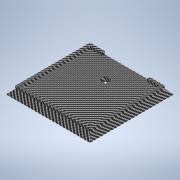
# Autodesk Inventor part: Base Plate
Saved by Autodesk Inventor 2021.1 (Build 251245010, 245A)
## iProperties
Created: 2020-11-23
Part Number: Base Plate
Material: CFRP
Document SubType Name: Modeling
Designer: elizh
Density: 1.43 g/cm^3
Appearance: Carbon Fiber
Author: elizh
Autodesk Inventor part; units mm, degrees
ref_plane "YZ Plane" through (0, 0, 0) normal (1, 0, 0) x (0, 1, 0)
ref_plane "XZ Plane" through (0, 0, 0) normal (0, 1, 0) x (-1, 0, 0)
ref_plane "XY Plane" through (0, 0, 0) normal (0, 0, 1) x (1, 0, 0)
sketch "Sketch1" plane through (0, 0, 0) normal (0, 1, 0) x (-1, 0, 0)
  line L0 (45, 45) -> (-45, 45)
  line L1 (-45, 45) -> (-45, -45)
  line L2 (-45, -45) -> (45, -45)
  line L3 (45, -45) -> (45, 45)
  line L4 (0, 0) -> (55.2623, 0) construction
  line L5 (0, 0) -> (0, -72.148) construction
  dimension "d0" = 90
  constraints: 12 end point, 2 horizontal, 2 parallel, 2 perpendicular, 1 vertical, 2 other
  measures "d0" distance of L2.end L0.start
extrude "Extrusion1" add sketch "Sketch1" along normal blind 5
chamfer "Chamfer2" distance 5 angle 45 4 edges at (-45, 5, 0) (0, 5, -45) (45, 5, 0) (0, 5, 45)
sketch "Sketch5" plane through (0, 5, 0) normal (0, 1, 0) x (1, 0, 0)
  line L0 (40, 40) -> (40, -40) projected
  line L1 (-40, 40) -> (40, 40) projected
  line L2 (-40, -40) -> (-40, 40) projected
  line L3 (40, -40) -> (-40, -40) projected
  line L4 (-37, -37) -> (37, -37)
  line L5 (37, -37) -> (37, 37)
  line L6 (-37, 37) -> (-37, -37)
  line L7 (-37, 37) -> (-24, 37)
  line L8 (-24, 37) -> (-24, 40)
  line L9 (-40, 40) -> (40, 40) projected
  line L10 (37, 37) -> (24, 37)
  line L11 (24, 37) -> (24, 40)
  point P0 (0, 0)
  dimension "d13" = 3
  dimension "d14" = 3
  dimension "d15" = 3
  dimension "d16" = 3
  dimension "d17" = 16
  dimension "d18" = 16
  constraints: 14 end point, 3 horizontal, 3 perpendicular, 2 point on line, 1 collinear, 1 parallel
  measures "d13" distance between parallel lines of L2 L6
  measures "d14" distance between parallel lines of L1 L7
  measures "d15" distance between parallel lines of L3 L4
  measures "d16" distance between parallel lines of L0 L5
  measures "d17" distance between parallel lines of L0 L11
  measures "d18" distance between parallel lines of L8 L2
extrude "Extrusion3" add sketch "Sketch5" along normal blind 3 contours L0 L3 L2 L1 L8 L7 L6 L4 L5 L10 L11
sketch "Sketch6" plane through (0, 5, 0) normal (0, 1, 0) x (1, 0, 0)
  line L0 (-3.5, 13) -> (3.5, 13)
  line L1 (3.5, 13) -> (3.5, 20)
  line L2 (3.5, 20) -> (-3.5, 20)
  line L3 (-3.5, 20) -> (-3.5, 13)
  line L4 (0, 0) -> (0, -11.2861) construction
  line L5 (-24, 40) -> (24, 40) projected
  dimension "d21" = 7
  dimension "d22" = 20
  constraints: 10 end point, 2 parallel, 2 perpendicular, 1 horizontal, 1 vertical, 1 other
  measures "d21" distance of L0.start L0.end
  measures "d22" distance between parallel lines of L5 L2
extrude "Extrusion4" cut sketch "Sketch6" against normal through all
equation "\"d14\" = d13"
equation "\"d15\" = d13"
equation "\"d16\" = d13"
equation "\"d18\" = d17"
body "Solid1"
